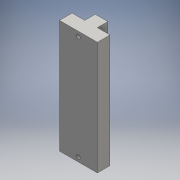
# Autodesk Inventor part: centerbeam
Saved by Autodesk Inventor 2016 (Build 200138000, 138)
## iProperties
Created: 2015-12-02
Part Number: centerbeam
Material: Generic
Document SubType Name: Modeling
Designer: hesaon
Density: 1 g/cm^3
Appearance: Default
Author: hesaon
Autodesk Inventor part; units mm, degrees
ref_plane "YZ Plane" through (0, 0, 0) normal (1, 0, 0) x (0, 1, 0)
ref_plane "XZ Plane" through (0, 0, 0) normal (0, 1, 0) x (-1, 0, 0)
ref_plane "XY Plane" through (0, 0, 0) normal (0, 0, 1) x (1, 0, 0)
sketch "Sketch1" plane through (0, 0, 0) normal (0, 0, 1) x (1, 0, 0)
  line L0 (0, 0) -> (36, 0)
  line L1 (36, 0) -> (36, 12)
  line L2 (36, 12) -> (24, 12)
  line L3 (24, 12) -> (24, 22)
  line L4 (24, 22) -> (12, 22)
  line L5 (12, 22) -> (12, 12)
  line L6 (12, 12) -> (0, 12)
  line L7 (0, 12) -> (0, 0)
  dimension "d0" = 36
  dimension "d1" = 12
  dimension "d2" = 12
  dimension "d3" = 10
  dimension "d4" = 12
  constraints: 16 end point, 6 perpendicular, 2 point on line, 1 horizontal
  measures "d0" distance of L0.start L0.end
  measures "d1" distance of L0.end L1.end
  measures "d2" distance of L1.end L2.end
  measures "d3" distance of L2.end L3.end
  measures "d4" distance of L3.end L4.end
extrude "Extrusion1" add sketch "Sketch1" along normal blind 108
sketch "Sketch2" plane through (0, 0, 0) normal (0, -1, 0) x (1, 0, 0)
  circle A0 centre (18, 4.5) radius 1.725
  line L0 (0, 0) -> (36, 0) projected
  line L1 (36, 0) -> (36, 108) projected
  circle A1 centre (18, 103.5) radius 1.725
  line L2 (0, 108) -> (36, 108) projected
  dimension "d7" = 3.45
  dimension "d8" = 4.5
  dimension "d9" = 18
  dimension "d10" = 3.45
  dimension "d11" = 18
  dimension "d12" = 4.5
  constraints: 2 centre point
  measures "d7" diameter of A0
  measures "d8" distance from line of L0 A0.centre
  measures "d9" distance from line of L1 A0.centre
  measures "d10" diameter of A1
  measures "d11" distance from line of L1 A1.centre
  measures "d12" distance from line of L2 A1.centre
extrude "Extrusion2" cut sketch "Sketch2" against normal blind 20
sketch "Sketch3" plane through (12, 22, 0) normal (0, 1, 0) x (1, 0, 0)
  circle A0 centre (6, -4.5) radius 1.725 projected
  circle A1 centre (6, -4.5) radius 3
  circle A2 centre (6, -103.5) radius 1.725 projected
  circle A3 centre (6, -103.5) radius 3
  point P0 (-12, 0)
  dimension "d15" = 6
  dimension "d16" = 6
  constraints: 2 centre point, 2 coincident
  measures "d15" diameter of A1
  measures "d16" diameter of A3
extrude "Extrusion3" cut sketch "Sketch3" against normal blind 2 contours A0 | A1 | A2 | A3
sketch "Sketch4" plane through (36, 0, 0) normal (1, 0, 0) x (0, 0, -1)
  line L0 (-108, 0) -> (-107.85, 0)
  line L1 (0, 0) -> (-108, 0) projected
  line L2 (-107.85, 0) -> (-107.85, 12)
  line L3 (0, 12) -> (-108, 12) projected
  line L4 (-108, 0) -> (-108, 12) projected
  line L5 (-108, 12) -> (-108, 0)
  line L6 (-108, 22) -> (-107.85, 22)
  line L7 (-107.85, 12) -> (-108, 12)
  line L8 (0, 0) -> (-0.15, 0)
  line L9 (-0.15, 0) -> (-0.15, 12)
  line L10 (-0.15, 12) -> (0, 12)
  line L11 (0, 12) -> (0, 0)
  line L12 (0, 22) -> (-0.15, 22)
  line L13 (-0.15, 12) -> (0, 12)
  dimension "d19" = 0.15
  dimension "d20" = 12
  dimension "d21" = 0.15
  dimension "d22" = 0.15
  constraints: 22 end point, 5 equal length, 3 horizontal, 3 point on line, 2 perpendicular
  measures "d19" distance of L0.start L0.end
  measures "d20" distance of L0.end L2.end
  measures "d21" distance of L3.end L2.end
  measures "d22" distance of L9.end L10.end
extrude "Extrusion4" cut sketch "Sketch4" against normal through all contours L4 L3 L2 L0 | L9 L3 L11 L1
sketch "Sketch5" plane through (24, 22, 108) normal (1, 0, 0) x (0, 0, -1)
  line L0 (108, -10) -> (108, 0) projected
  line L1 (108, 0) -> (0, 0) projected
  line L2 (108, -10) -> (107.85, -10)
  line L3 (107.85, -10) -> (107.85, 0)
  line L4 (107.85, 0) -> (108, 0)
  line L5 (108, 0) -> (108, -10)
  line L6 (0.15, -10) -> (0, -10) projected
  line L7 (0, -10) -> (0, 0) projected
  line L8 (0.15, -10) -> (0, -10)
  line L9 (0, -10) -> (0, 0)
  line L10 (0, 0) -> (0.15, 0)
  line L11 (0.15, 0) -> (0.15, -10)
  point P0 (108, -22)
  dimension "d25" = 0.15
  constraints: 16 end point, 4 parallel, 2 horizontal, 2 perpendicular, 1 point on line
  measures "d25" distance of L3.end L4.end
extrude "Extrusion5" cut sketch "Sketch5" against normal through all
body "Solid1"
